Autodesk Fusion 360 part; units mm, degrees
(part 4 of 25)
  arc A1244 (33.5788, 10.6144) -> (33.6296, 10.6144) centre (33.6042, 10.6144) ccw
  arc A1245 (33.2147, 10.8994) -> (33.2147, 10.8486) centre (33.2147, 10.874) ccw
  arc A1246 (32.4278, 11.3271) -> (32.4438, 11.2789) centre (32.4358, 11.303) ccw
  line L381 (32.4358, 10.2249) -> (32.4358, 10.874)
  line L382 (35.6898, 8.9408) -> (35.6898, 9.7197)
  line L383 (32.4358, 11.303) -> (33.6042, 11.6925)
  line L384 (32.9551, 10.2249) -> (32.4358, 10.2249)
  arc A1247 (35.7547, 10.8994) -> (35.7547, 10.8486) centre (35.7547, 10.874) ccw
  arc A1248 (36.0793, 9.3049) -> (36.0793, 9.3557) centre (36.0793, 9.3303) ccw
  arc A1249 (35.8846, 10.8486) -> (35.8846, 10.8994) centre (35.8846, 10.874) ccw
  line L385 (33.3446, 10.874) -> (33.2147, 10.874)
  arc A1250 (32.9805, 10.6144) -> (32.9297, 10.6144) centre (32.9551, 10.6144) ccw
  arc A1251 (32.4358, 10.2503) -> (32.4358, 10.1995) centre (32.4358, 10.2249) ccw
  line L386 (55.2958, 13.5292) -> (55.2958, 13.7889)
  arc A1252 (33.5393, 9.3049) -> (33.5393, 9.3557) centre (33.5393, 9.3303) ccw
  arc A1253 (55.5554, 13.295) -> (55.5554, 13.2442) centre (55.5554, 13.2696) ccw
  arc A1254 (33.2147, 10.8486) -> (33.2147, 10.8994) centre (33.2147, 10.874) ccw
  arc A1255 (33.2147, 10.874) -> (32.9551, 10.6144) centre (33.2147, 10.6144) ccw
  arc A1256 (33.3446, 10.8994) -> (33.3446, 10.8486) centre (33.3446, 10.874) ccw
  arc A1257 (35.7152, 9.7197) -> (35.6644, 9.7197) centre (35.6898, 9.7197) ccw
  line L387 (55.2958, 14.2658) -> (56.4642, 14.2658)
  arc A1258 (32.4612, 10.874) -> (32.4104, 10.874) centre (32.4358, 10.874) ccw
  arc A1259 (55.2958, 14.2912) -> (55.2958, 14.2404) centre (55.2958, 14.2658) ccw
  arc A1260 (33.6122, 11.6684) -> (33.5962, 11.7166) centre (33.6042, 11.6925) ccw
  arc A1261 (32.4104, 10.2249) -> (32.4612, 10.2249) centre (32.4358, 10.2249) ccw
  arc A1262 (33.5962, 11.6684) -> (33.6122, 11.7166) centre (33.6042, 11.6925) ccw
  arc A1263 (55.3212, 13.7889) -> (55.2704, 13.7889) centre (55.2958, 13.7889) ccw
  arc A1264 (36.1188, 10.6144) -> (36.1696, 10.6144) centre (36.1442, 10.6144) ccw
  arc A1265 (55.2958, 13.5292) -> (55.5554, 13.2696) centre (55.5554, 13.5292) ccw
  arc A1266 (33.6296, 10.6144) -> (33.5788, 10.6144) centre (33.6042, 10.6144) ccw
  arc A1267 (33.3446, 10.8486) -> (33.3446, 10.8994) centre (33.3446, 10.874) ccw
  arc A1268 (32.9297, 10.6144) -> (32.9805, 10.6144) centre (32.9551, 10.6144) ccw
  arc A1269 (36.1442, 10.6144) -> (35.8846, 10.874) centre (35.8846, 10.6144) ccw
  arc A1270 (36.1188, 10.2249) -> (36.1696, 10.2249) centre (36.1442, 10.2249) ccw
  arc A1271 (55.5554, 13.2442) -> (55.5554, 13.295) centre (55.5554, 13.2696) ccw
  arc A1272 (33.6042, 10.6144) -> (33.3446, 10.874) centre (33.3446, 10.6144) ccw
  arc A1273 (32.7604, 9.3557) -> (32.7604, 9.3049) centre (32.7604, 9.3303) ccw
  arc A1274 (35.8846, 10.8994) -> (35.8846, 10.8486) centre (35.8846, 10.874) ccw
  line L388 (35.4951, 10.6144) -> (35.4951, 10.2249)
  line L389 (34.9758, 10.2249) -> (34.9758, 10.874)
  arc A1275 (37.5412, 9.2004) -> (37.4904, 9.2004) centre (37.5158, 9.2004) ccw
  arc A1276 (37.5412, 9.5899) -> (37.4904, 9.5899) centre (37.5158, 9.5899) ccw
  arc A1277 (37.8404, 12.0283) -> (37.5158, 11.7037) centre (37.8404, 11.7037) ccw
  arc A1278 (35.4697, 10.2249) -> (35.5205, 10.2249) centre (35.4951, 10.2249) ccw
  arc A1279 (35.5205, 10.6144) -> (35.4697, 10.6144) centre (35.4951, 10.6144) ccw
  line L390 (38.0351, 9.5899) -> (38.6842, 9.5899)
  arc A1280 (38.0351, 9.6153) -> (38.0351, 9.5645) centre (38.0351, 9.5899) ccw
  arc A1281 (38.6842, 10.1346) -> (38.6842, 10.1854) centre (38.6842, 10.16) ccw
  line L391 (38.6842, 9.5899) -> (38.6842, 9.2004)
  arc A1282 (37.5158, 11.4046) -> (37.5158, 11.3538) centre (37.5158, 11.3792) ccw
  arc A1283 (38.6842, 11.7037) -> (38.3596, 12.0283) centre (38.3596, 11.7037) ccw
  arc A1284 (38.3596, 12.0029) -> (38.3596, 12.0537) centre (38.3596, 12.0283) ccw
  line L392 (37.5158, 9.2004) -> (37.5158, 9.5899)
  line L393 (37.5158, 10.16) -> (38.6842, 10.8091)
  arc A1285 (38.0097, 9.3952) -> (38.0605, 9.3952) centre (38.0351, 9.3952) ccw
  arc A1286 (34.9504, 10.2249) -> (35.0012, 10.2249) centre (34.9758, 10.2249) ccw
  arc A1287 (38.0605, 9.5899) -> (38.0097, 9.5899) centre (38.0351, 9.5899) ccw
  arc A1288 (37.5035, 10.1822) -> (37.5281, 10.1378) centre (37.5158, 10.16) ccw
  arc A1289 (35.7547, 10.874) -> (35.4951, 10.6144) centre (35.7547, 10.6144) ccw
  arc A1290 (36.1522, 11.6684) -> (36.1362, 11.7166) centre (36.1442, 11.6925) ccw
  arc A1291 (34.9838, 12.106) -> (34.9678, 12.0578) centre (34.9758, 12.0819) ccw
  arc A1292 (37.5158, 10.8345) -> (37.5158, 10.7837) centre (37.5158, 10.8091) ccw
  arc A1293 (38.4246, 8.9408) -> (38.6842, 9.2004) centre (38.4246, 9.2004) ccw
  arc A1294 (37.4904, 9.2004) -> (37.5412, 9.2004) centre (37.5158, 9.2004) ccw
  arc A1295 (38.6842, 10.7837) -> (38.6842, 10.8345) centre (38.6842, 10.8091) ccw
  arc A1296 (38.6842, 9.5645) -> (38.6842, 9.6153) centre (38.6842, 9.5899) ccw
  arc A1297 (37.5158, 10.1854) -> (37.5158, 10.1346) centre (37.5158, 10.16) ccw
  arc A1298 (38.6965, 10.7869) -> (38.6719, 10.8313) centre (38.6842, 10.8091) ccw
  line L394 (34.9758, 11.303) -> (36.1442, 11.6925)
  arc A1299 (34.9678, 11.3271) -> (34.9838, 11.2789) centre (34.9758, 11.303) ccw
  arc A1300 (37.7754, 8.9154) -> (37.7754, 8.9662) centre (37.7754, 8.9408) ccw
  arc A1301 (35.4697, 10.6144) -> (35.5205, 10.6144) centre (35.4951, 10.6144) ccw
  arc A1302 (38.7096, 9.5899) -> (38.6588, 9.5899) centre (38.6842, 9.5899) ccw
  arc A1303 (38.4246, 8.9154) -> (38.4246, 8.9662) centre (38.4246, 8.9408) ccw
  arc A1304 (37.7754, 8.9662) -> (37.7754, 8.9154) centre (37.7754, 8.9408) ccw
  line L395 (37.5158, 11.3792) -> (37.5158, 11.7037)
  line L396 (38.6842, 10.8091) -> (37.5158, 10.8091)
  arc A1305 (35.4951, 10.1995) -> (35.4951, 10.2503) centre (35.4951, 10.2249) ccw
  line L397 (38.6842, 10.16) -> (37.5158, 10.16)
  line L398 (38.0351, 9.3952) -> (38.0351, 9.5899)
  arc A1306 (35.0012, 10.874) -> (34.9504, 10.874) centre (34.9758, 10.874) ccw
  arc A1307 (37.4904, 11.3792) -> (37.5412, 11.3792) centre (37.5158, 11.3792) ccw
  arc A1308 (37.5158, 9.2004) -> (37.7754, 8.9408) centre (37.7754, 9.2004) ccw
  arc A1309 (37.8404, 12.0029) -> (37.8404, 12.0537) centre (37.8404, 12.0283) ccw
  arc A1310 (37.5412, 11.7037) -> (37.4904, 11.7037) centre (37.5158, 11.7037) ccw
  arc A1311 (34.9758, 10.2503) -> (34.9758, 10.1995) centre (34.9758, 10.2249) ccw
  arc A1312 (38.7096, 9.2004) -> (38.6588, 9.2004) centre (38.6842, 9.2004) ccw
  arc A1313 (38.6842, 11.3538) -> (38.6842, 11.4046) centre (38.6842, 11.3792) ccw
  arc A1314 (37.4904, 11.7037) -> (37.5412, 11.7037) centre (37.5158, 11.7037) ccw
  line L399 (37.8404, 12.0283) -> (38.3596, 12.0283)
  arc A1315 (38.6588, 11.7037) -> (38.7096, 11.7037) centre (38.6842, 11.7037) ccw
  arc A1316 (38.6588, 11.3792) -> (38.7096, 11.3792) centre (38.6842, 11.3792) ccw
  line L400 (29.1451, 28.6399) -> (29.7942, 28.6399)
  line L401 (36.1442, 11.6925) -> (34.9758, 12.0819)
  arc A1317 (38.3596, 12.0537) -> (38.3596, 12.0029) centre (38.3596, 12.0283) ccw
  line L402 (38.6842, 11.3792) -> (37.5158, 11.3792)
  arc A1318 (37.8404, 12.0537) -> (37.8404, 12.0029) centre (37.8404, 12.0283) ccw
  arc A1319 (36.1362, 11.6684) -> (36.1522, 11.7166) centre (36.1442, 11.6925) ccw
  arc A1320 (38.6588, 9.2004) -> (38.7096, 9.2004) centre (38.6842, 9.2004) ccw
  line L403 (35.4951, 10.2249) -> (34.9758, 10.2249)
  arc A1321 (38.4246, 8.9662) -> (38.4246, 8.9154) centre (38.4246, 8.9408) ccw
  line L404 (38.4246, 8.9408) -> (37.7754, 8.9408)
  arc A1322 (51.1175, 9.6224) -> (51.0667, 9.6224) centre (51.0921, 9.6224) ccw
  arc A1323 (48.2115, 10.7198) -> (48.1786, 10.6811) centre (48.1951, 10.7005) ccw
  arc A1324 (50.1904, 10.5382) -> (50.2412, 10.5382) centre (50.2158, 10.5382) ccw
  arc A1325 (48.1951, 10.7005) -> (47.9679, 10.7978) centre (47.968, 10.4841) ccw
  arc A1326 (50.7605, 10.5382) -> (50.7097, 10.5382) centre (50.7351, 10.5382) ccw
  arc A1327 (50.7097, 10.2785) -> (50.7605, 10.2785) centre (50.7351, 10.2785) ccw
  line L405 (53.9242, 8.9408) -> (52.7558, 9.3303)
  arc A1328 (47.9679, 10.8232) -> (47.9679, 10.7724) centre (47.9679, 10.7978) ccw
  arc A1329 (48.1767, 10.6829) -> (48.2135, 10.718) centre (48.1951, 10.7005) ccw
  arc A1330 (48.8277, 10.1294) -> (48.8607, 10.1681) centre (48.8442, 10.1488) ccw
  line L406 (51.3842, 8.9408) -> (50.2158, 9.3303)
  line L407 (48.8442, 10.1487) -> (48.8442, 10.7978)
  arc A1331 (51.4096, 10.4733) -> (51.3588, 10.4733) centre (51.3842, 10.4733) ccw
  arc A1332 (53.9322, 9.6956) -> (53.9162, 9.7438) centre (53.9242, 9.7197) ccw
  arc A1333 (53.6575, 9.6224) -> (53.6067, 9.6224) centre (53.6321, 9.6224) ccw
  line L408 (53.6646, 10.1487) -> (53.6646, 10.7978)
  line L409 (52.7558, 10.4084) -> (53.6646, 10.1487)
  arc A1334 (51.3588, 10.1487) -> (51.4096, 10.1487) centre (51.3842, 10.1487) ccw
  line L410 (50.2158, 10.1487) -> (50.2158, 10.5382)
  arc A1335 (53.6576, 10.1243) -> (53.6715, 10.1731) centre (53.6646, 10.1487) ccw
  arc A1336 (48.8188, 10.1487) -> (48.8696, 10.1487) centre (48.8442, 10.1487) ccw
  line L411 (50.7351, 10.5382) -> (50.7351, 10.2785)
  arc A1337 (53.9162, 8.9167) -> (53.9322, 8.9649) centre (53.9242, 8.9408) ccw
  arc A1338 (50.7097, 10.5382) -> (50.7605, 10.5382) centre (50.7351, 10.5382) ccw
  line L412 (52.7558, 9.3303) -> (53.9242, 9.7197)
  arc A1339 (51.3842, 10.4733) -> (50.7351, 10.4733) centre (51.0597, 10.4733) ccw
  line L413 (48.1951, 10.7005) -> (48.8442, 10.1487)
  arc A1340 (48.8696, 10.7978) -> (48.8188, 10.7978) centre (48.8442, 10.7978) ccw
  arc A1341 (50.2078, 9.3544) -> (50.2238, 9.3062) centre (50.2158, 9.3303) ccw
  arc A1342 (50.7351, 10.5382) -> (50.2158, 10.5382) centre (50.4755, 10.5382) ccw
  line L414 (38.6842, 11.7037) -> (38.6842, 11.3792)
  arc A1343 (51.3762, 8.9167) -> (51.3922, 8.9649) centre (51.3842, 8.9408) ccw
  arc A1344 (51.3588, 10.4733) -> (51.4096, 10.4733) centre (51.3842, 10.4733) ccw
  arc A1345 (52.7638, 9.3544) -> (52.7478, 9.3062) centre (52.7558, 9.3303) ccw
  arc A1346 (50.1904, 10.1487) -> (50.2412, 10.1487) centre (50.2158, 10.1487) ccw
  arc A1347 (52.7478, 9.3544) -> (52.7638, 9.3062) centre (52.7558, 9.3303) ccw
  arc A1348 (51.3922, 9.6956) -> (51.3762, 9.7438) centre (51.3842, 9.7197) ccw
  line L415 (53.6321, 9.6224) -> (53.6321, 9.0382)
  arc A1349 (53.6067, 9.0382) -> (53.6575, 9.0382) centre (53.6321, 9.0382) ccw
  arc A1350 (50.7097, 10.4733) -> (50.7605, 10.4733) centre (50.7351, 10.4733) ccw
  arc A1351 (29.1451, 28.6653) -> (29.1451, 28.6145) centre (29.1451, 28.6399) ccw
  arc A1352 (47.7012, 10.5057) -> (47.6504, 10.5057) centre (47.6758, 10.5057) ccw
  arc A1353 (47.9276, 10.1245) -> (47.9433, 10.1729) centre (47.9355, 10.1487) ccw
  line L416 (51.0921, 9.6224) -> (51.0921, 9.0382)
  arc A1354 (51.0667, 9.0382) -> (51.1175, 9.0382) centre (51.0921, 9.0382) ccw
  arc A1355 (50.2238, 9.3544) -> (50.2078, 9.3062) centre (50.2158, 9.3303) ccw
  arc A1356 (47.6758, 10.5057) -> (47.9354, 10.1487) centre (48.051, 10.5057) ccw
  arc A1357 (29.5346, 27.9908) -> (29.7942, 28.2504) centre (29.5346, 28.2504) ccw
  line L417 (50.2158, 9.3303) -> (51.3842, 9.7197)
  arc A1358 (47.6504, 10.5057) -> (47.7012, 10.5057) centre (47.6758, 10.5057) ccw
  line L418 (51.3842, 10.1487) -> (51.3842, 10.4733)
  arc A1359 (50.2412, 10.5382) -> (50.1904, 10.5382) centre (50.2158, 10.5382) ccw
  arc A1360 (27.3304, 20.6657) -> (27.3812, 20.6657) centre (27.3558, 20.6657) ccw
  arc A1361 (41.2242, 20.2946) -> (41.2242, 20.3454) centre (41.2242, 20.32) ccw
  line L419 (40.5751, 19.7499) -> (41.2242, 19.7499)
  line L420 (25.9842, 19.1008) -> (24.8158, 19.4903)
  arc A1362 (23.0547, 21.034) -> (22.7951, 20.7744) centre (23.0547, 20.7744) ccw
  arc A1363 (27.6479, 20.9324) -> (27.6479, 20.9832) centre (27.6479, 20.9578) ccw
  arc A1364 (27.8915, 20.8798) -> (27.8586, 20.8411) centre (27.8751, 20.8605) ccw
  arc A1365 (40.3804, 22.2137) -> (40.3804, 22.1629) centre (40.3804, 22.1883) ccw
  line L421 (25.0754, 20.3087) -> (24.8158, 20.6333)
  arc A1366 (41.1988, 21.5392) -> (41.2496, 21.5392) centre (41.2242, 21.5392) ccw
  arc A1367 (41.2242, 21.5138) -> (41.2242, 21.5646) centre (41.2242, 21.5392) ccw
  line L422 (31.0642, 19.1008) -> (29.8958, 19.4903)
  arc A1368 (41.2242, 21.8637) -> (40.8996, 22.1883) centre (40.8996, 21.8637) ccw
  arc A1369 (25.9588, 20.3087) -> (26.0096, 20.3087) centre (25.9842, 20.3087) ccw
  arc A1370 (40.0558, 21.5646) -> (40.0558, 21.5138) centre (40.0558, 21.5392) ccw
  arc A1371 (40.0304, 21.8637) -> (40.0812, 21.8637) centre (40.0558, 21.8637) ccw
  line L423 (28.5242, 20.3087) -> (28.5242, 20.9578)
  arc A1372 (24.8078, 19.5144) -> (24.8238, 19.4662) centre (24.8158, 19.4903) ccw
  line L424 (22.7951, 20.7744) -> (22.7951, 20.3849)
  arc A1373 (25.9842, 20.6079) -> (25.9842, 20.6587) centre (25.9842, 20.6333) ccw
  arc A1374 (27.3812, 20.6657) -> (27.3304, 20.6657) centre (27.3558, 20.6657) ccw
  arc A1375 (29.9038, 19.5144) -> (29.8878, 19.4662) centre (29.8958, 19.4903) ccw
  arc A1376 (25.9922, 19.8556) -> (25.9762, 19.9038) centre (25.9842, 19.8797) ccw
  arc A1377 (28.4988, 20.3087) -> (28.5496, 20.3087) centre (28.5242, 20.3087) ccw
  arc A1378 (28.5162, 19.0767) -> (28.5322, 19.1249) centre (28.5242, 19.1008) ccw
  arc A1379 (40.0558, 20.3454) -> (40.0558, 20.2946) centre (40.0558, 20.32) ccw
  arc A1380 (28.5322, 19.8556) -> (28.5162, 19.9038) centre (28.5242, 19.8797) ccw
  arc A1381 (27.8567, 20.8429) -> (27.8935, 20.878) centre (27.8751, 20.8605) ccw
  arc A1382 (41.1988, 21.8637) -> (41.2496, 21.8637) centre (41.2242, 21.8637) ccw
  line L425 (25.6921, 19.7824) -> (25.6921, 19.1982)
  arc A1383 (41.2242, 20.9437) -> (41.2242, 20.9945) centre (41.2242, 20.9691) ccw
  arc A1384 (25.9762, 19.0767) -> (25.9922, 19.1249) centre (25.9842, 19.1008) ccw
  arc A1385 (24.8238, 19.5144) -> (24.8078, 19.4662) centre (24.8158, 19.4903) ccw
  arc A1386 (40.8996, 22.2137) -> (40.8996, 22.1629) centre (40.8996, 22.1883) ccw
  arc A1387 (23.0547, 21.0086) -> (23.0547, 21.0594) centre (23.0547, 21.034) ccw
  arc A1388 (27.6479, 20.9832) -> (27.6479, 20.9324) centre (27.6479, 20.9578) ccw
  arc A1389 (28.2067, 19.1982) -> (28.2575, 19.1982) centre (28.2321, 19.1982) ccw
  arc A1390 (41.2496, 21.8637) -> (41.1988, 21.8637) centre (41.2242, 21.8637) ccw
  arc A1391 (25.7175, 19.7824) -> (25.6667, 19.7824) centre (25.6921, 19.7824) ccw
  line L426 (27.8751, 20.8605) -> (28.5242, 20.3087)
  arc A1392 (28.5077, 20.2894) -> (28.5407, 20.3281) centre (28.5242, 20.3087) ccw
  arc A1393 (28.2575, 19.7824) -> (28.2067, 19.7824) centre (28.2321, 19.7824) ccw
  arc A1394 (31.0562, 19.0767) -> (31.0722, 19.1249) centre (31.0642, 19.1008) ccw
  arc A1395 (25.0556, 20.2928) -> (25.0953, 20.3246) centre (25.0755, 20.3087) ccw
  arc A1396 (23.3793, 19.4649) -> (23.3793, 19.5157) centre (23.3793, 19.4903) ccw
  line L427 (24.8158, 20.6333) -> (25.9842, 20.6333)
  line L428 (25.9842, 20.3087) -> (25.9842, 20.9578)
  arc A1397 (40.3804, 22.1629) -> (40.3804, 22.2137) centre (40.3804, 22.1883) ccw
  arc A1398 (24.8158, 20.6587) -> (24.8158, 20.6079) centre (24.8158, 20.6333) ccw
  line L429 (28.5242, 19.1008) -> (27.3558, 19.4903)
  arc A1399 (23.0152, 19.8797) -> (22.9644, 19.8797) centre (22.9898, 19.8797) ccw
  line L430 (41.2242, 21.5392) -> (40.0558, 21.5392)
  arc A1400 (27.3638, 19.5144) -> (27.3478, 19.4662) centre (27.3558, 19.4903) ccw
  arc A1401 (40.0812, 21.8637) -> (40.0304, 21.8637) centre (40.0558, 21.8637) ccw
  line L431 (40.3804, 22.1883) -> (40.8996, 22.1883)
  arc A1402 (25.6667, 19.1982) -> (25.7175, 19.1982) centre (25.6921, 19.1982) ccw
  arc A1403 (24.8356, 20.6491) -> (24.796, 20.6174) centre (24.8158, 20.6333) ccw
  line L432 (27.3558, 19.4903) -> (28.5242, 19.8797)
  arc A1404 (41.2365, 20.9469) -> (41.2119, 20.9913) centre (41.2242, 20.9691) ccw
  arc A1405 (26.0096, 20.9578) -> (25.9588, 20.9578) centre (25.9842, 20.9578) ccw
  line L433 (28.2321, 19.7824) -> (28.2321, 19.1982)
  arc A1406 (27.8751, 20.8605) -> (27.6479, 20.9578) centre (27.648, 20.6441) ccw
  line L434 (24.8158, 19.4903) -> (25.9842, 19.8797)
  arc A1407 (27.6479, 20.9578) -> (27.3558, 20.6657) centre (27.6479, 20.6657) ccw
  line L435 (32.7604, 20.931) -> (33.0849, 20.931)
  arc A1408 (32.7604, 20.9564) -> (32.7604, 20.9056) centre (32.7604, 20.931) ccw
  arc A1409 (31.0896, 20.6333) -> (31.0388, 20.6333) centre (31.0642, 20.6333) ccw
  arc A1410 (32.7604, 20.2565) -> (32.7604, 20.3073) centre (32.7604, 20.2819) ccw
  arc A1411 (33.6042, 20.4117) -> (33.0849, 20.931) centre (33.0849, 20.4117) ccw
  arc A1412 (30.3897, 20.4385) -> (30.4405, 20.4385) centre (30.4151, 20.4385) ccw
  arc A1413 (32.4612, 19.4254) -> (32.4104, 19.4254) centre (32.4358, 19.4254) ccw
  arc A1414 (40.3804, 22.1883) -> (40.0558, 21.8637) centre (40.3804, 21.8637) ccw
  arc A1415 (27.6076, 20.2845) -> (27.6233, 20.3329) centre (27.6155, 20.3087) ccw
  arc A1416 (35.3004, 19.7499) -> (34.9758, 19.4254) centre (35.3004, 19.4253) ccw
  arc A1417 (34.9504, 19.1008) -> (35.0012, 19.1008) centre (34.9758, 19.1008) ccw
  arc A1418 (30.7467, 19.1982) -> (30.7975, 19.1982) centre (30.7721, 19.1982) ccw
  arc A1419 (40.8996, 22.1629) -> (40.8996, 22.2137) centre (40.8996, 22.1883) ccw
  arc A1420 (27.3478, 19.5144) -> (27.3638, 19.4662) centre (27.3558, 19.4903) ccw
  arc A1421 (32.4358, 19.1262) -> (32.4358, 19.0754) centre (32.4358, 19.1008) ccw
  arc A1422 (32.4104, 19.4254) -> (32.4612, 19.4254) centre (32.4358, 19.4254) ccw
  arc A1423 (32.8253, 20.2819) -> (33.0849, 20.5415) centre (32.8253, 20.5415) ccw
  line L436 (33.6042, 19.1008) -> (32.4358, 19.1008)
  arc A1424 (29.8878, 19.5144) -> (29.9038, 19.4662) centre (29.8958, 19.4903) ccw
  arc A1425 (32.8253, 20.3073) -> (32.8253, 20.2565) centre (32.8253, 20.2819) ccw
  arc A1426 (33.1103, 20.5415) -> (33.0595, 20.5415) centre (33.0849, 20.5415) ccw
  arc A1427 (32.8253, 20.2565) -> (32.8253, 20.3073) centre (32.8253, 20.2819) ccw
  line L437 (40.0558, 21.5392) -> (40.0558, 21.8637)
  arc A1428 (31.0642, 20.6333) -> (30.4151, 20.6333) centre (30.7396, 20.6333) ccw
  line L438 (31.0642, 20.3087) -> (31.0642, 20.6333)
  line L439 (33.6042, 19.4254) -> (33.6042, 19.1008)
  arc A1429 (27.3558, 20.6657) -> (27.6154, 20.3087) centre (27.731, 20.6657) ccw
  line L440 (41.2242, 21.8637) -> (41.2242, 21.5392)
  line L441 (29.8958, 19.4903) -> (31.0642, 19.8797)
  line L442 (30.4151, 20.6982) -> (30.4151, 20.4385)
  arc A1430 (31.0388, 20.6333) -> (31.0896, 20.6333) centre (31.0642, 20.6333) ccw
  arc A1431 (30.4405, 20.6982) -> (30.3897, 20.6982) centre (30.4151, 20.6982) ccw
  arc A1432 (33.6042, 19.4254) -> (33.2796, 19.7499) centre (33.2796, 19.4253) ccw
  arc A1433 (33.0595, 20.5415) -> (33.1103, 20.5415) centre (33.0849, 20.5415) ccw
  arc A1434 (32.7604, 19.7499) -> (32.4358, 19.4254) centre (32.7604, 19.4253) ccw
  arc A1435 (40.0304, 21.5392) -> (40.0812, 21.5392) centre (40.0558, 21.5392) ccw
  arc A1436 (30.4151, 20.6982) -> (29.8958, 20.6982) centre (30.1554, 20.6982) ccw
  arc A1437 (32.7604, 20.3073) -> (32.7604, 20.2565) centre (32.7604, 20.2819) ccw
  line L443 (32.7604, 19.7499) -> (33.2796, 19.7499)
  arc A1438 (33.5788, 19.1008) -> (33.6296, 19.1008) centre (33.6042, 19.1008) ccw
  line L444 (34.9758, 19.1008) -> (34.9758, 19.4254)
  arc A1439 (31.0722, 19.8556) -> (31.0562, 19.9038) centre (31.0642, 19.8797) ccw
  arc A1440 (30.3897, 20.6982) -> (30.4405, 20.6982) centre (30.4151, 20.6982) ccw
  arc A1441 (28.5496, 20.9578) -> (28.4988, 20.9578) centre (28.5242, 20.9578) ccw
  arc A1442 (33.2796, 19.7753) -> (33.2796, 19.7245) centre (33.2796, 19.7499) ccw
  arc A1443 (29.8704, 20.6982) -> (29.9212, 20.6982) centre (29.8958, 20.6982) ccw
  arc A1444 (32.4104, 19.1008) -> (32.4612, 19.1008) centre (32.4358, 19.1008) ccw
  arc A1445 (32.7604, 19.7245) -> (32.7604, 19.7753) centre (32.7604, 19.7499) ccw
  arc A1446 (33.0849, 20.9056) -> (33.0849, 20.9564) centre (33.0849, 20.931) ccw
  arc A1447 (29.8704, 20.3087) -> (29.9212, 20.3087) centre (29.8958, 20.3087) ccw
  arc A1448 (32.7604, 19.7753) -> (32.7604, 19.7245) centre (32.7604, 19.7499) ccw
  arc A1449 (30.7975, 19.7824) -> (30.7467, 19.7824) centre (30.7721, 19.7824) ccw
  line L445 (29.8958, 20.3087) -> (29.8958, 20.6982)
  line L446 (30.7721, 19.7824) -> (30.7721, 19.1982)
  arc A1450 (33.2796, 19.7245) -> (33.2796, 19.7753) centre (33.2796, 19.7499) ccw
  arc A1451 (31.0388, 20.3087) -> (31.0896, 20.3087) centre (31.0642, 20.3087) ccw
  arc A1452 (30.3897, 20.6333) -> (30.4405, 20.6333) centre (30.4151, 20.6333) ccw
  arc A1453 (32.7604, 20.931) -> (32.7604, 20.2819) centre (32.7604, 20.6065) ccw
  arc A1454 (35.0012, 19.4254) -> (34.9504, 19.4254) centre (34.9758, 19.4254) ccw
  line L447 (33.0849, 20.931) -> (33.0849, 20.5415)
  arc A1455 (29.9212, 20.6982) -> (29.8704, 20.6982) centre (29.8958, 20.6982) ccw
  line L448 (32.4358, 19.1008) -> (32.4358, 19.4254)
  arc A1456 (32.7604, 20.9056) -> (32.7604, 20.9564) centre (32.7604, 20.931) ccw
  arc A1457 (33.6296, 19.4254) -> (33.5788, 19.4254) centre (33.6042, 19.4254) ccw
  line L449 (36.1442, 20.2819) -> (36.1442, 20.931)
  arc A1458 (35.1269, 21.9995) -> (35.1492, 21.9538) centre (35.138, 21.9767) ccw
  arc A1459 (34.9956, 20.6223) -> (34.956, 20.5906) centre (34.9758, 20.6065) ccw
  arc A1460 (35.2513, 22.0289) -> (35.2196, 21.9893) centre (35.2355, 22.0091) ccw
  arc A1461 (35.1492, 21.5451) -> (35.1269, 21.4994) centre (35.138, 21.5223) ccw
  arc A1462 (35.9737, 21.5463) -> (35.9902, 21.4982) centre (35.9819, 21.5222) ccw
  arc A1463 (35.9902, 22.0007) -> (35.9737, 21.9526) centre (35.9819, 21.9767) ccw
  arc A1464 (38.2552, 25.0613) -> (38.2044, 25.0613) centre (38.2298, 25.0613) ccw
  line L450 (36.1442, 19.4254) -> (36.1442, 19.1008)
  arc A1465 (33.1103, 20.931) -> (33.0595, 20.931) centre (33.0849, 20.931) ccw
  arc A1466 (36.1188, 19.1008) -> (36.1696, 19.1008) centre (36.1442, 19.1008) ccw
  arc A1467 (35.8196, 19.7753) -> (35.8196, 19.7245) centre (35.8196, 19.7499) ccw
  arc A1468 (38.2552, 23.7659) -> (38.2044, 23.7659) centre (38.2298, 23.7659) ccw
  line L451 (38.2298, 24.2824) -> (38.2298, 25.0613)
  arc A1469 (33.5788, 19.4254) -> (33.6296, 19.4254) centre (33.6042, 19.4254) ccw
  arc A1470 (34.9758, 19.1262) -> (34.9758, 19.0754) centre (34.9758, 19.1008) ccw
  arc A1471 (36.1442, 19.0754) -> (36.1442, 19.1262) centre (36.1442, 19.1008) ccw
  line L452 (38.2298, 20.3962) -> (38.2298, 21.1751)
  line L453 (35.3004, 19.7499) -> (35.8196, 19.7499)
  arc A1472 (35.56, 21.4503) -> (35.56, 21.3995) centre (35.56, 21.4249) ccw
  arc A1473 (36.1188, 20.2819) -> (36.1696, 20.2819) centre (36.1442, 20.2819) ccw
  arc A1474 (35.8687, 21.47) -> (35.9004, 21.5096) centre (35.8845, 21.4898) ccw
  arc A1475 (38.2552, 19.8797) -> (38.2044, 19.8797) centre (38.2298, 19.8797) ccw
  arc A1476 (38.2044, 24.2824) -> (38.2552, 24.2824) centre (38.2298, 24.2824) ccw
  line L454 (38.2298, 22.987) -> (38.2298, 23.7659)
  arc A1477 (33.0849, 20.9564) -> (33.0849, 20.9056) centre (33.0849, 20.931) ccw
  arc A1478 (35.56, 22.074) -> (35.1381, 21.9766) centre (35.5601, 21.1113) ccw
  arc A1479 (35.0012, 21.7494) -> (34.9504, 21.7494) centre (34.9758, 21.7494) ccw
  arc A1480 (33.6042, 19.0754) -> (33.6042, 19.1262) centre (33.6042, 19.1008) ccw
  arc A1481 (34.9758, 20.6319) -> (34.9758, 20.5811) centre (34.9758, 20.6065) ccw
  arc A1482 (33.5788, 20.4117) -> (33.6296, 20.4117) centre (33.6042, 20.4117) ccw
  line L455 (34.9758, 20.6065) -> (36.1442, 20.6065)
  arc A1483 (34.9504, 21.7494) -> (35.0012, 21.7494) centre (34.9758, 21.7494) ccw
  arc A1484 (38.2044, 20.3962) -> (38.2552, 20.3962) centre (38.2298, 20.3962) ccw
  arc A1485 (36.1442, 21.7494) -> (35.9819, 21.9766) centre (35.904, 21.7494) ccw
  arc A1486 (35.1381, 21.9766) -> (34.9758, 21.7494) centre (35.216, 21.7494) ccw
  arc A1487 (36.1696, 21.7494) -> (36.1188, 21.7494) centre (36.1442, 21.7494) ccw
  arc A1488 (36.1442, 20.5811) -> (36.1442, 20.6319) centre (36.1442, 20.6065) ccw
  arc A1489 (35.1463, 21.9526) -> (35.1298, 22.0007) centre (35.138, 21.9766) ccw
  arc A1490 (35.9931, 21.4994) -> (35.9708, 21.5451) centre (35.982, 21.5223) ccw
  line L456 (32.8253, 20.2819) -> (32.7604, 20.2819)
  arc A1491 (35.56, 21.4249) -> (35.9819, 21.5223) centre (35.5599, 22.3876) ccw
  arc A1492 (36.1442, 19.4254) -> (35.8196, 19.7499) centre (35.8196, 19.4253) ccw
  arc A1493 (35.3004, 19.7753) -> (35.3004, 19.7245) centre (35.3004, 19.7499) ccw
  arc A1494 (35.56, 22.0994) -> (35.56, 22.0486) centre (35.56, 22.074) ccw
  line L457 (38.2298, 19.1008) -> (38.2298, 19.8797)
  arc A1495 (34.9504, 19.4254) -> (35.0012, 19.4254) centre (34.9758, 19.4254) ccw
  arc A1496 (36.1696, 20.931) -> (36.1188, 20.931) centre (36.1442, 20.931) ccw
  line L458 (76.7842, 35.6108) -> (75.6158, 36.0003)
  arc A1497 (35.9819, 21.5223) -> (36.1442, 21.7494) centre (35.9041, 21.7494) ccw
  arc A1498 (35.8196, 19.7245) -> (35.8196, 19.7753) centre (35.8196, 19.7499) ccw
  arc A1499 (36.1188, 21.7494) -> (36.1696, 21.7494) centre (36.1442, 21.7494) ccw
  arc A1500 (35.56, 22.0486) -> (35.56, 22.0994) centre (35.56, 22.074) ccw
  arc A1501 (75.6238, 36.0244) -> (75.6078, 35.9762) centre (75.6158, 36.0003) ccw
  arc A1502 (35.1381, 21.5223) -> (35.56, 21.4249) centre (35.5601, 22.3876) ccw
  arc A1503 (34.9758, 21.7494) -> (35.1381, 21.5223) centre (35.2159, 21.7494) ccw
  arc A1504 (35.1298, 21.4982) -> (35.1463, 21.5463) centre (35.1381, 21.5222) ccw
  line L459 (38.2298, 21.6916) -> (38.2298, 22.4705)
  arc A1505 (35.9819, 21.9766) -> (35.56, 22.074) centre (35.5599, 21.1113) ccw
  arc A1506 (36.1696, 19.4254) -> (36.1188, 19.4254) centre (36.1442, 19.4254) ccw
  arc A1507 (38.2044, 19.1008) -> (38.2552, 19.1008) centre (38.2298, 19.1008) ccw
  arc A1508 (35.9708, 21.9538) -> (35.9931, 21.9995) centre (35.9819, 21.9767) ccw
  arc A1509 (36.1188, 19.4254) -> (36.1696, 19.4254) centre (36.1442, 19.4254) ccw
  line L460 (36.1442, 19.1008) -> (34.9758, 19.1008)
  arc A1510 (75.9404, 40.6301) -> (75.6158, 40.3056) centre (75.9404, 40.3055) ccw
  arc A1511 (75.5904, 40.3056) -> (75.6412, 40.3056) centre (75.6158, 40.3056) ccw
  arc A1512 (75.6228, 37.1028) -> (75.6088, 37.0539) centre (75.6158, 37.0784) ccw
  arc A1513 (75.6412, 40.3056) -> (75.5904, 40.3056) centre (75.6158, 40.3056) ccw
  arc A1514 (75.7335, 39.407) -> (75.6928, 39.4374) centre (75.7132, 39.4222) ccw
  arc A1515 (76.4596, 40.6555) -> (76.4596, 40.6047) centre (76.4596, 40.6301) ccw
  arc A1516 (76.4992, 36.8187) -> (76.55, 36.8187) centre (76.5246, 36.8187) ccw
  arc A1517 (76.2649, 37.2985) -> (76.2649, 37.2477) centre (76.2649, 37.2731) ccw
  line L461 (75.6158, 36.0003) -> (76.7842, 36.3897)
  arc A1518 (75.9404, 40.6047) -> (75.9404, 40.6555) centre (75.9404, 40.6301) ccw
  line L462 (76.914, 37.9123) -> (75.486, 38.4316)
  arc A1519 (76.0803, 39.0124) -> (76.1249, 38.9881) centre (76.1026, 39.0003) ccw
  arc A1520 (38.2552, 21.1751) -> (38.2044, 21.1751) centre (38.2298, 21.1751) ccw
  line L463 (76.2649, 37.2731) -> (76.7842, 37.2731)
  arc A1521 (76.55, 37.4678) -> (76.4992, 37.4678) centre (76.5246, 37.4678) ccw
  arc A1522 (75.6078, 36.0244) -> (75.6238, 35.9762) centre (75.6158, 36.0003) ccw
  arc A1523 (75.8754, 38.8705) -> (76.1026, 39.0003) centre (75.8754, 39.1342) ccw
  arc A1524 (76.7588, 39.2275) -> (76.8096, 39.2275) centre (76.7842, 39.2275) ccw
  arc A1525 (76.8096, 39.2275) -> (76.7588, 39.2275) centre (76.7842, 39.2275) ccw
  arc A1526 (35.3004, 19.7245) -> (35.3004, 19.7753) centre (35.3004, 19.7499) ccw
  line L464 (76.2974, 39.3573) -> (76.1026, 39.0003)
  arc A1527 (38.2044, 21.6916) -> (38.2552, 21.6916) centre (38.2298, 21.6916) ccw
  arc A1528 (76.6219, 38.838) -> (76.7842, 39.2275) centre (76.2357, 39.2275) ccw
  arc A1529 (35.2156, 20.266) -> (35.2553, 20.2978) centre (35.2355, 20.2819) ccw
  arc A1530 (75.8754, 38.8959) -> (75.8754, 38.8451) centre (75.8754, 38.8705) ccw
  line L465 (76.7842, 39.981) -> (75.6158, 39.981)
  line L466 (75.6158, 41.4867) -> (76.7842, 41.8761)
  line L467 (75.6158, 37.0784) -> (76.5246, 36.8187)
  arc A1531 (76.7922, 41.852) -> (76.7762, 41.9002) centre (76.7842, 41.8761) ccw
  arc A1532 (75.4947, 38.4555) -> (75.4773, 38.4077) centre (75.486, 38.4316) ccw
  arc A1533 (75.6158, 39.1301) -> (75.8754, 38.8705) centre (75.8754, 39.1301) ccw
  arc A1534 (76.9053, 37.8884) -> (76.9227, 37.9362) centre (76.914, 37.9123) ccw
  arc A1535 (75.6412, 39.1301) -> (75.5904, 39.1301) centre (75.6158, 39.1301) ccw
  line L468 (35.8846, 21.4898) -> (35.2354, 22.0091)
  arc A1536 (38.2044, 22.987) -> (38.2552, 22.987) centre (38.2298, 22.987) ccw
  arc A1537 (76.4596, 40.6047) -> (76.4596, 40.6555) centre (76.4596, 40.6301) ccw
  arc A1538 (75.6158, 40.0064) -> (75.6158, 39.9556) centre (75.6158, 39.981) ccw
  arc A1539 (35.56, 21.3995) -> (35.56, 21.4503) centre (35.56, 21.4249) ccw
  arc A1540 (76.5246, 39.4871) -> (76.2974, 39.3573) centre (76.5246, 39.2234) ccw
  arc A1541 (76.7842, 39.2275) -> (76.5246, 39.4871) centre (76.5246, 39.2275) ccw
  arc A1542 (76.7922, 36.3656) -> (76.7762, 36.4138) centre (76.7842, 36.3897) ccw
  arc A1543 (75.9404, 40.6555) -> (75.9404, 40.6047) centre (75.9404, 40.6301) ccw
  line L469 (35.2354, 20.2819) -> (34.9758, 20.6065)
  arc A1544 (75.7132, 39.4222) -> (75.6158, 39.1301) centre (76.1026, 39.1301) ccw
  arc A1545 (76.7842, 39.9556) -> (76.7842, 40.0064) centre (76.7842, 39.981) ccw
  arc A1546 (76.7588, 40.3056) -> (76.8096, 40.3056) centre (76.7842, 40.3056) ccw
  arc A1547 (76.2755, 39.3702) -> (76.3193, 39.3444) centre (76.2974, 39.3573) ccw
  line L470 (76.7842, 40.3056) -> (76.7842, 39.981)
  arc A1548 (75.5904, 39.1301) -> (75.6412, 39.1301) centre (75.6158, 39.1301) ccw
  arc A1549 (76.604, 38.856) -> (76.6398, 38.82) centre (76.6219, 38.838) ccw
  line L471 (76.5246, 36.8187) -> (76.5246, 37.4678)
  arc A1550 (76.5246, 39.5125) -> (76.5246, 39.4617) centre (76.5246, 39.4871) ccw
  arc A1551 (76.7842, 37.2477) -> (76.7842, 37.2985) centre (76.7842, 37.2731) ccw
  arc A1552 (75.6078, 41.5108) -> (75.6238, 41.4626) centre (75.6158, 41.4867) ccw
  line L472 (75.6158, 39.981) -> (75.6158, 40.3056)
  line L473 (75.9404, 40.6301) -> (76.4596, 40.6301)
  arc A1553 (38.2552, 22.4705) -> (38.2044, 22.4705) centre (38.2298, 22.4705) ccw
  arc A1554 (75.5904, 39.981) -> (75.6412, 39.981) centre (75.6158, 39.981) ccw
  arc A1555 (76.4667, 35.7082) -> (76.5175, 35.7082) centre (76.4921, 35.7082) ccw
  arc A1556 (76.7762, 35.5867) -> (76.7922, 35.6349) centre (76.7842, 35.6108) ccw
  arc A1557 (76.5176, 36.7943) -> (76.5315, 36.8431) centre (76.5246, 36.8187) ccw
  arc A1558 (76.5175, 36.2924) -> (76.4667, 36.2924) centre (76.4921, 36.2924) ccw
  line L474 (76.4921, 36.2924) -> (76.4921, 35.7082)
  arc A1559 (75.8754, 38.8451) -> (75.8754, 38.8959) centre (75.8754, 38.8705) ccw
  arc A1560 (76.7762, 41.0731) -> (76.7922, 41.1213) centre (76.7842, 41.0972) ccw
  arc A1561 (76.4667, 41.1946) -> (76.5175, 41.1946) centre (76.4921, 41.1946) ccw
  arc A1562 (79.3496, 40.1992) -> (79.2988, 40.1992) centre (79.3242, 40.1992) ccw
  arc A1563 (79.3242, 39.2275) -> (79.0646, 39.4871) centre (79.0646, 39.2275) ccw
  arc A1564 (78.6497, 36.8187) -> (78.7005, 36.8187) centre (78.6751, 36.8187) ccw
  arc A1565 (76.7842, 40.3056) -> (76.4596, 40.6301) centre (76.4596, 40.3055) ccw
  arc A1566 (76.8096, 40.3056) -> (76.7588, 40.3056) centre (76.7842, 40.3056) ccw
  arc A1567 (78.9347, 37.4932) -> (78.9347, 37.4424) centre (78.9347, 37.4678) ccw
  arc A1568 (79.4453, 37.8884) -> (79.4627, 37.9362) centre (79.454, 37.9123) ccw
  arc A1569 (79.0646, 39.965) -> (79.0646, 39.9142) centre (79.0646, 39.9396) ccw
  line L475 (78.1558, 36.8187) -> (78.1558, 37.4678)
  line L476 (79.0321, 36.2924) -> (79.0321, 35.7082)
  arc A1570 (79.3322, 36.3656) -> (79.3162, 36.4138) centre (79.3242, 36.3897) ccw
  arc A1571 (78.9347, 37.4678) -> (78.6751, 37.2082) centre (78.9347, 37.2082) ccw
  arc A1572 (78.6751, 36.7933) -> (78.6751, 36.8441) centre (78.6751, 36.8187) ccw
  arc A1573 (79.0646, 37.4932) -> (79.0646, 37.4424) centre (79.0646, 37.4678) ccw
  arc A1574 (79.2988, 37.2082) -> (79.3496, 37.2082) centre (79.3242, 37.2082) ccw
  line L477 (78.8374, 39.3573) -> (78.6426, 39.0003)
  line L478 (79.3242, 40.4589) -> (79.3242, 40.1992)
  arc A1575 (76.5175, 41.7788) -> (76.4667, 41.7788) centre (76.4921, 41.7788) ccw
  arc A1576 (76.1245, 38.9874) -> (76.0808, 39.0132) centre (76.1026, 39.0003) ccw
  arc A1577 (75.6238, 41.5108) -> (75.6078, 41.4626) centre (75.6158, 41.4867) ccw
  arc A1578 (78.8597, 39.3451) -> (78.8151, 39.3695) centre (78.8374, 39.3573) ccw
  arc A1579 (79.3242, 37.2082) -> (79.0646, 37.4678) centre (79.0646, 37.2082) ccw
  arc A1580 (78.1478, 36.0244) -> (78.1638, 35.9762) centre (78.1558, 36.0003) ccw
  line L479 (78.6751, 36.8187) -> (78.1558, 36.8187)
  line L480 (78.1558, 36.0003) -> (79.3242, 36.3897)
  arc A1581 (78.0347, 38.4555) -> (78.0173, 38.4077) centre (78.026, 38.4316) ccw
  arc A1582 (79.0646, 39.9396) -> (79.3242, 40.1992) centre (79.0646, 40.1992) ccw
  line L481 (79.0646, 37.4678) -> (78.9347, 37.4678)
  arc A1583 (76.5246, 39.4617) -> (76.5246, 39.5125) centre (76.5246, 39.4871) ccw
  arc A1584 (79.1619, 38.838) -> (79.3242, 39.2275) centre (78.7757, 39.2275) ccw
  line L482 (79.0646, 39.9396) -> (78.4154, 39.9396)
  arc A1585 (78.1304, 39.1301) -> (78.1812, 39.1301) centre (78.1558, 39.1301) ccw
  arc A1586 (79.0646, 37.4424) -> (79.0646, 37.4932) centre (79.0646, 37.4678) ccw
  line L483 (76.4921, 41.7788) -> (76.4921, 41.1946)
  arc A1587 (79.144, 38.856) -> (79.1798, 38.82) centre (79.1619, 38.838) ccw
  arc A1588 (79.3162, 35.5867) -> (79.3322, 35.6349) centre (79.3242, 35.6108) ccw
  arc A1589 (78.4154, 38.8451) -> (78.4154, 38.8959) centre (78.4154, 38.8705) ccw
  arc A1590 (76.7588, 39.981) -> (76.8096, 39.981) centre (76.7842, 39.981) ccw
  arc A1591 (79.0575, 36.2924) -> (79.0067, 36.2924) centre (79.0321, 36.2924) ccw
  arc A1592 (78.1304, 36.8187) -> (78.1812, 36.8187) centre (78.1558, 36.8187) ccw
  arc A1593 (78.1812, 39.1301) -> (78.1304, 39.1301) centre (78.1558, 39.1301) ccw
  arc A1594 (79.0646, 39.4617) -> (79.0646, 39.5125) centre (79.0646, 39.4871) ccw
  arc A1595 (79.2988, 40.1992) -> (79.3496, 40.1992) centre (79.3242, 40.1992) ccw
  line L484 (78.6751, 37.2082) -> (78.6751, 36.8187)
  arc A1596 (78.2532, 39.4222) -> (78.1558, 39.1301) centre (78.6426, 39.1301) ccw
  arc A1597 (76.3197, 39.3451) -> (76.2751, 39.3695) centre (76.2974, 39.3573) ccw
  arc A1598 (78.1812, 37.4678) -> (78.1304, 37.4678) centre (78.1558, 37.4678) ccw
  arc A1599 (78.1638, 36.0244) -> (78.1478, 35.9762) centre (78.1558, 36.0003) ccw
  arc A1600 (79.0646, 39.4871) -> (78.8374, 39.3573) centre (79.0646, 39.2234) ccw
  arc A1601 (79.3496, 37.2082) -> (79.2988, 37.2082) centre (79.3242, 37.2082) ccw
  arc A1602 (78.6497, 37.2082) -> (78.7005, 37.2082) centre (78.6751, 37.2082) ccw
  arc A1603 (78.1558, 39.1301) -> (78.4154, 38.8705) centre (78.4154, 39.1301) ccw
  arc A1604 (79.0067, 35.7082) -> (79.0575, 35.7082) centre (79.0321, 35.7082) ccw
  arc A1605 (79.3496, 39.2275) -> (79.2988, 39.2275) centre (79.3242, 39.2275) ccw
  arc A1606 (79.2988, 36.8187) -> (79.3496, 36.8187) centre (79.3242, 36.8187) ccw
  line L485 (79.454, 37.9123) -> (78.026, 38.4316)
  arc A1607 (79.2988, 39.2275) -> (79.3496, 39.2275) centre (79.3242, 39.2275) ccw
  arc A1608 (78.6645, 38.9874) -> (78.6208, 39.0132) centre (78.6427, 39.0003) ccw
  arc A1609 (78.2735, 39.407) -> (78.2328, 39.4374) centre (78.2532, 39.4222) ccw
  line L486 (76.7842, 41.0972) -> (75.6158, 41.4867)
  arc A1610 (78.4154, 38.8705) -> (78.6426, 39.0003) centre (78.4154, 39.1342) ccw
  arc A1611 (78.9347, 37.4424) -> (78.9347, 37.4932) centre (78.9347, 37.4678) ccw
  line L487 (79.3242, 36.8187) -> (79.3242, 37.2082)
  arc A1612 (81.8642, 39.6437) -> (81.5396, 39.9683) centre (81.5396, 39.6437) ccw
  arc A1613 (81.8642, 38.0746) -> (81.8642, 38.1254) centre (81.8642, 38.1) ccw
  arc A1614 (80.6704, 37.1404) -> (80.7212, 37.1404) centre (80.6958, 37.1404) ccw
  arc A1615 (78.7005, 37.2082) -> (78.6497, 37.2082) centre (78.6751, 37.2082) ccw
  arc A1616 (81.8896, 37.1404) -> (81.8388, 37.1404) centre (81.8642, 37.1404) ccw
  line L488 (81.6046, 36.8808) -> (80.9554, 36.8808)
  arc A1617 (81.8896, 37.5299) -> (81.8388, 37.5299) centre (81.8642, 37.5299) ccw
  arc A1618 (81.8642, 39.2938) -> (81.8642, 39.3446) centre (81.8642, 39.3192) ccw
  line L489 (79.3242, 35.6108) -> (78.1558, 36.0003)
  arc A1619 (78.1558, 36.8441) -> (78.1558, 36.7933) centre (78.1558, 36.8187) ccw
  arc A1620 (78.8155, 39.3702) -> (78.8593, 39.3444) centre (78.8374, 39.3573) ccw
  arc A1621 (81.8896, 39.6437) -> (81.8388, 39.6437) centre (81.8642, 39.6437) ccw
  arc A1622 (78.1558, 40.1992) -> (78.4154, 39.9396) centre (78.4154, 40.1992) ccw
  arc A1623 (81.1897, 37.3352) -> (81.2405, 37.3352) centre (81.2151, 37.3352) ccw
  arc A1624 (81.8765, 38.7269) -> (81.8519, 38.7713) centre (81.8642, 38.7491) ccw
  arc A1625 (81.5396, 39.9937) -> (81.5396, 39.9429) centre (81.5396, 39.9683) ccw
  arc A1626 (81.8642, 37.5045) -> (81.8642, 37.5553) centre (81.8642, 37.5299) ccw
  arc A1627 (79.2988, 40.9358) -> (79.3496, 40.9358) centre (79.3242, 40.9358) ccw
  line L490 (78.1558, 40.9358) -> (79.3242, 40.9358)
  arc A1628 (80.6958, 38.7745) -> (80.6958, 38.7237) centre (80.6958, 38.7491) ccw
  arc A1629 (78.1304, 40.1992) -> (78.1812, 40.1992) centre (78.1558, 40.1992) ccw
  arc A1630 (80.7212, 37.1404) -> (80.6704, 37.1404) centre (80.6958, 37.1404) ccw
  line L491 (80.6958, 39.3192) -> (80.6958, 39.6437)
  arc A1631 (79.3496, 41.455) -> (79.2988, 41.455) centre (79.3242, 41.455) ccw
  arc A1632 (78.1812, 40.4589) -> (78.1304, 40.4589) centre (78.1558, 40.4589) ccw
  arc A1633 (81.8642, 38.7237) -> (81.8642, 38.7745) centre (81.8642, 38.7491) ccw
  arc A1634 (80.6835, 38.1222) -> (80.7081, 38.0778) centre (80.6958, 38.1) ccw
  arc A1635 (81.2405, 37.5299) -> (81.1897, 37.5299) centre (81.2151, 37.5299) ccw
  arc A1636 (81.6046, 36.8808) -> (81.8642, 37.1404) centre (81.6046, 37.1404) ccw
  arc A1637 (78.4154, 39.9142) -> (78.4154, 39.965) centre (78.4154, 39.9396) ccw
  arc A1638 (80.6704, 39.6437) -> (80.7212, 39.6437) centre (80.6958, 39.6437) ccw
  line L492 (81.8642, 39.6437) -> (81.8642, 39.3192)
  arc A1639 (81.2151, 37.5553) -> (81.2151, 37.5045) centre (81.2151, 37.5299) ccw
  line L493 (81.8642, 39.3192) -> (80.6958, 39.3192)
  line L494 (81.8642, 38.7491) -> (80.6958, 38.7491)
  arc A1640 (80.9554, 36.8554) -> (80.9554, 36.9062) centre (80.9554, 36.8808) ccw
  line L495 (80.6958, 38.1) -> (81.8642, 38.7491)
  arc A1641 (78.1558, 40.9612) -> (78.1558, 40.9104) centre (78.1558, 40.9358) ccw
  arc A1642 (79.3242, 40.9104) -> (79.3242, 40.9612) centre (79.3242, 40.9358) ccw
  arc A1643 (81.6046, 36.8554) -> (81.6046, 36.9062) centre (81.6046, 36.8808) ccw
  line L496 (81.8642, 38.1) -> (80.6958, 38.1)
  line L497 (78.1558, 40.1992) -> (78.1558, 40.4589)
  arc A1644 (80.7212, 39.6437) -> (80.6704, 39.6437) centre (80.6958, 39.6437) ccw
  arc A1645 (81.0204, 39.9683) -> (80.6958, 39.6437) centre (81.0204, 39.6437) ccw
  arc A1646 (81.8388, 37.1404) -> (81.8896, 37.1404) centre (81.8642, 37.1404) ccw
  line L498 (81.2151, 37.3352) -> (81.2151, 37.5299)
  arc A1647 (81.8388, 39.3192) -> (81.8896, 39.3192) centre (81.8642, 39.3192) ccw
  arc A1648 (79.0646, 39.9142) -> (79.0646, 39.965) centre (79.0646, 39.9396) ccw
  arc A1649 (81.6046, 36.9062) -> (81.6046, 36.8554) centre (81.6046, 36.8808) ccw
  arc A1650 (78.4154, 38.8959) -> (78.4154, 38.8451) centre (78.4154, 38.8705) ccw
  arc A1651 (79.0646, 39.5125) -> (79.0646, 39.4617) centre (79.0646, 39.4871) ccw
  arc A1652 (78.6203, 39.0124) -> (78.6649, 38.9881) centre (78.6426, 39.0003) ccw
  arc A1653 (80.6958, 37.1404) -> (80.9554, 36.8808) centre (80.9554, 37.1404) ccw
  arc A1654 (73.8152, 37.6597) -> (73.7644, 37.6597) centre (73.7898, 37.6597) ccw
  arc A1655 (78.4154, 39.965) -> (78.4154, 39.9142) centre (78.4154, 39.9396) ccw
  line L499 (79.3242, 40.9358) -> (79.3242, 41.455)
  arc A1656 (79.3496, 40.4589) -> (79.2988, 40.4589) centre (79.3242, 40.4589) ccw
  arc A1657 (80.7212, 37.5299) -> (80.6704, 37.5299) centre (80.6958, 37.5299) ccw
  line L500 (73.7898, 36.8808) -> (73.7898, 37.6597)
  arc A1658 (81.8388, 39.6437) -> (81.8896, 39.6437) centre (81.8642, 39.6437) ccw
  arc A1659 (80.6958, 39.3446) -> (80.6958, 39.2938) centre (80.6958, 39.3192) ccw
  line L501 (81.8642, 37.5299) -> (81.8642, 37.1404)
  arc A1660 (81.5396, 39.9429) -> (81.5396, 39.9937) centre (81.5396, 39.9683) ccw
  arc A1661 (4.0462, 47.7012) -> (3.9954, 47.7012) centre (4.0208, 47.7012) ccw
  arc A1662 (5.5307, 46.5074) -> (5.5307, 46.5582) centre (5.5307, 46.5328) ccw
  arc A1663 (80.6958, 38.1254) -> (80.6958, 38.0746) centre (80.6958, 38.1) ccw
  line L502 (80.6958, 37.1404) -> (80.6958, 37.5299)
  line L503 (73.0758, 38.1649) -> (73.0758, 38.814)
  line L504 (73.0758, 39.243) -> (74.2442, 39.6325)
  arc A1664 (73.5697, 38.1649) -> (73.6205, 38.1649) centre (73.5951, 38.1649) ccw
  arc A1665 (74.2188, 38.5544) -> (74.2696, 38.5544) centre (74.2442, 38.5544) ccw
  arc A1666 (2.8448, 47.7266) -> (2.8448, 47.6758) centre (2.8448, 47.7012) ccw
  line L505 (3.1694, 47.0521) -> (2.8448, 47.0521)
  arc A1667 (73.0758, 38.1903) -> (73.0758, 38.1395) centre (73.0758, 38.1649) ccw
  arc A1668 (73.8547, 38.8394) -> (73.8547, 38.7886) centre (73.8547, 38.814) ccw
  arc A1669 (73.9846, 38.7886) -> (73.9846, 38.8394) centre (73.9846, 38.814) ccw
  arc A1670 (3.1694, 47.0521) -> (3.1694, 47.7012) centre (3.1694, 47.3767) ccw
  arc A1671 (3.1694, 47.7266) -> (3.1694, 47.6758) centre (3.1694, 47.7012) ccw
  arc A1672 (2.8448, 47.0775) -> (2.8448, 47.0267) centre (2.8448, 47.0521) ccw
  line L506 (74.2442, 39.6325) -> (73.0758, 40.0219)
  arc A1673 (73.4004, 37.2957) -> (73.4004, 37.2449) centre (73.4004, 37.2703) ccw
  arc A1674 (81.0204, 39.9429) -> (81.0204, 39.9937) centre (81.0204, 39.9683) ccw
  arc A1675 (4.5401, 47.6758) -> (4.5401, 47.7266) centre (4.5401, 47.7012) ccw
  arc A1676 (4.4103, 47.1565) -> (4.4103, 47.2073) centre (4.4103, 47.1819) ccw
  arc A1677 (2.8702, 47.7012) -> (2.8194, 47.7012) centre (2.8448, 47.7012) ccw
  arc A1678 (3.1694, 47.0775) -> (3.1694, 47.0267) centre (3.1694, 47.0521) ccw
  line L507 (5.0114, 46.5328) -> (5.5307, 46.5328)
  arc A1679 (78.1812, 40.1992) -> (78.1304, 40.1992) centre (78.1558, 40.1992) ccw
  arc A1680 (4.0208, 47.7266) -> (4.0208, 47.6758) centre (4.0208, 47.7012) ccw
  line L508 (4.5401, 46.5328) -> (4.0208, 46.5328)
  line L509 (74.1793, 37.2703) -> (73.4004, 37.2703)
  arc A1681 (73.9846, 38.8394) -> (73.9846, 38.7886) centre (73.9846, 38.814) ccw
  arc A1682 (74.2362, 39.6084) -> (74.2522, 39.6566) centre (74.2442, 39.6325) ccw
  arc A1683 (73.8547, 38.7886) -> (73.8547, 38.8394) centre (73.8547, 38.814) ccw
  arc A1684 (80.6704, 39.3192) -> (80.7212, 39.3192) centre (80.6958, 39.3192) ccw
  arc A1685 (81.0204, 39.9937) -> (81.0204, 39.9429) centre (81.0204, 39.9683) ccw
  arc A1686 (73.1012, 38.814) -> (73.0504, 38.814) centre (73.0758, 38.814) ccw
  arc A1687 (3.9954, 46.5328) -> (4.0462, 46.5328) centre (4.0208, 46.5328) ccw
  line L510 (4.0208, 46.5328) -> (4.0208, 47.7012)
  arc A1688 (3.257, 47.0634) -> (3.2115, 47.0407) centre (3.2343, 47.0521) ccw
  arc A1689 (74.2442, 38.5544) -> (73.9846, 38.814) centre (73.9846, 38.5544) ccw
  arc A1690 (3.4712, 46.5214) -> (3.5166, 46.5442) centre (3.4939, 46.5328) ccw
  arc A1691 (73.0838, 40.046) -> (73.0678, 39.9978) centre (73.0758, 40.0219) ccw
  arc A1692 (3.1694, 47.0267) -> (3.1694, 47.0775) centre (3.1694, 47.0521) ccw
  arc A1693 (2.8194, 46.5328) -> (2.8702, 46.5328) centre (2.8448, 46.5328) ccw
  line L511 (74.2442, 38.1649) -> (74.2442, 38.5544)
  line L512 (4.0208, 47.7012) -> (4.5401, 47.7012)
  arc A1694 (74.1793, 37.2449) -> (74.1793, 37.2957) centre (74.1793, 37.2703) ccw
  arc A1695 (74.2188, 38.1649) -> (74.2696, 38.1649) centre (74.2442, 38.1649) ccw
  arc A1696 (73.8547, 38.814) -> (73.5951, 38.5544) centre (73.8547, 38.5544) ccw
  arc A1697 (4.5401, 46.5074) -> (4.5401, 46.5582) centre (4.5401, 46.5328) ccw
  line L513 (81.0204, 39.9683) -> (81.5396, 39.9683)
  line L514 (2.8448, 47.7012) -> (3.1694, 47.7012)
  arc A1698 (80.9554, 36.9062) -> (80.9554, 36.8554) centre (80.9554, 36.8808) ccw
  line L515 (81.2151, 37.5299) -> (81.8642, 37.5299)
  arc A1699 (4.0208, 47.2073) -> (4.0208, 47.1565) centre (4.0208, 47.1819) ccw
  arc A1700 (5.0368, 47.7012) -> (4.986, 47.7012) centre (5.0114, 47.7012) ccw
  arc A1701 (74.2696, 38.5544) -> (74.2188, 38.5544) centre (74.2442, 38.5544) ccw
  arc A1702 (73.5697, 38.5544) -> (73.6205, 38.5544) centre (73.5951, 38.5544) ccw
  arc A1703 (73.6205, 38.5544) -> (73.5697, 38.5544) centre (73.5951, 38.5544) ccw
  arc A1704 (74.2522, 39.6084) -> (74.2362, 39.6566) centre (74.2442, 39.6325) ccw
  arc A1705 (5.0114, 46.5582) -> (5.0114, 46.5074) centre (5.0114, 46.5328) ccw
  line L516 (4.0208, 47.1819) -> (4.4103, 47.1819)
  arc A1706 (73.5951, 38.1395) -> (73.5951, 38.1903) centre (73.5951, 38.1649) ccw
  arc A1707 (73.0504, 38.1649) -> (73.1012, 38.1649) centre (73.0758, 38.1649) ccw
  line L517 (3.4939, 46.5328) -> (3.2343, 47.0521)
  arc A1708 (4.0208, 46.5582) -> (4.0208, 46.5074) centre (4.0208, 46.5328) ccw
  arc A1709 (21.0058, 53.8311) -> (21.0058, 53.7803) centre (21.0058, 53.8057) ccw
  arc A1710 (22.1865, 55.0605) -> (22.1619, 55.1049) centre (22.1742, 55.0827) ccw
  arc A1711 (18.8327, 52.4482) -> (18.8835, 52.4482) centre (18.8581, 52.4482) ccw
  arc A1712 (18.8835, 52.6429) -> (18.8327, 52.6429) centre (18.8581, 52.6429) ccw
  arc A1713 (5.9941, 46.8503) -> (5.9941, 46.7995) centre (5.9941, 46.8249) ccw
  arc A1714 (7.4084, 47.1641) -> (7.4499, 47.1348) centre (7.4292, 47.1495) ccw
  line L518 (5.0114, 47.7012) -> (5.0114, 46.5328)
  line L519 (73.9846, 38.814) -> (73.8547, 38.814)
  line L520 (22.1742, 52.8913) -> (21.0058, 53.2807)
  arc A1715 (20.9804, 53.6758) -> (21.0312, 53.6758) centre (21.0058, 53.6758) ccw
  arc A1716 (21.0058, 55.1081) -> (21.0058, 55.0573) centre (21.0058, 55.0827) ccw
  arc A1717 (5.8726, 46.5408) -> (5.9208, 46.5248) centre (5.8967, 46.5328) ccw
  line L521 (18.8581, 52.4482) -> (18.8581, 52.6429)
  arc A1718 (22.1742, 54.4082) -> (22.1742, 54.459) centre (22.1742, 54.4336) ccw
  line L522 (19.2476, 51.9938) -> (18.5984, 51.9938)
  arc A1719 (7.4084, 47.1348) -> (7.4499, 47.1641) centre (7.4291, 47.1494) ccw
  line L523 (21.0058, 52.5018) -> (22.1742, 52.8913)
  arc A1720 (7.8394, 47.6866) -> (7.7979, 47.7158) centre (7.8187, 47.7012) ccw
  line L524 (7.4292, 46.5328) -> (7.4292, 47.1495)
  arc A1721 (7.4546, 47.1495) -> (7.4038, 47.1495) centre (7.4292, 47.1495) ccw
  arc A1722 (22.1742, 55.0573) -> (22.1742, 55.1081) centre (22.1742, 55.0827) ccw
  arc A1723 (18.3642, 52.2534) -> (18.3134, 52.2534) centre (18.3388, 52.2534) ccw
  arc A1724 (19.4818, 52.2534) -> (19.5326, 52.2534) centre (19.5072, 52.2534) ccw
  arc A1725 (19.5326, 52.2534) -> (19.4818, 52.2534) centre (19.5072, 52.2534) ccw
  arc A1726 (18.3642, 52.6429) -> (18.3134, 52.6429) centre (18.3388, 52.6429) ccw
  arc A1727 (22.1996, 53.9355) -> (22.1488, 53.9355) centre (22.1742, 53.9355) ccw
  line L525 (7.4292, 47.1495) -> (7.8187, 47.7012)
  arc A1728 (4.986, 46.5328) -> (5.0368, 46.5328) centre (5.0114, 46.5328) ccw
  arc A1729 (20.9935, 54.4558) -> (21.0181, 54.4114) centre (21.0058, 54.4336) ccw
  arc A1730 (21.0138, 53.3048) -> (20.9978, 53.2566) centre (21.0058, 53.2807) ccw
  arc A1731 (19.2476, 51.9684) -> (19.2476, 52.0192) centre (19.2476, 51.9938) ccw
  arc A1732 (6.3103, 47.7092) -> (6.2621, 47.6932) centre (6.2862, 47.7012) ccw
  arc A1733 (19.2476, 51.9938) -> (19.5072, 52.2534) centre (19.2476, 52.2534) ccw
  line L526 (73.5951, 38.5544) -> (73.5951, 38.1649)
  line L527 (73.5951, 38.1649) -> (73.0758, 38.1649)
  arc A1734 (18.3134, 52.2534) -> (18.3642, 52.2534) centre (18.3388, 52.2534) ccw
  line L528 (6.5783, 46.8249) -> (5.9941, 46.8249)
  line L529 (7.0397, 47.7012) -> (7.4292, 47.1495)
  line L530 (18.3388, 52.2534) -> (18.3388, 52.6429)
  arc A1735 (21.0312, 53.9355) -> (20.9804, 53.9355) centre (21.0058, 53.9355) ccw
  arc A1736 (18.8581, 52.6683) -> (18.8581, 52.6175) centre (18.8581, 52.6429) ccw
  line L531 (18.8581, 52.6429) -> (19.5072, 52.6429)
  arc A1737 (22.1488, 53.6758) -> (22.1996, 53.6758) centre (22.1742, 53.6758) ccw
  line L532 (22.1742, 55.0827) -> (21.0058, 55.0827)
  line L533 (21.0058, 53.8057) -> (22.1742, 53.8057)
  line L534 (5.8967, 46.5328) -> (6.2862, 47.7012)
  line L535 (21.0058, 53.6758) -> (21.0058, 53.9355)
  arc A1738 (3.1694, 47.6758) -> (3.1694, 47.7266) centre (3.1694, 47.7012) ccw
  line L536 (19.5072, 52.6429) -> (19.5072, 52.2534)
  arc A1739 (20.9978, 52.5259) -> (21.0138, 52.4777) centre (21.0058, 52.5018) ccw
  arc A1740 (73.7644, 36.8808) -> (73.8152, 36.8808) centre (73.7898, 36.8808) ccw
  arc A1741 (19.2476, 52.0192) -> (19.2476, 51.9684) centre (19.2476, 51.9938) ccw
  arc A1742 (6.5783, 46.7995) -> (6.5783, 46.8503) centre (6.5783, 46.8249) ccw
  line L537 (2.8448, 46.5328) -> (2.8448, 47.7012)
  arc A1743 (18.5984, 52.0192) -> (18.5984, 51.9684) centre (18.5984, 51.9938) ccw
  line L538 (6.2862, 47.7012) -> (6.6757, 46.5328)
  arc A1744 (21.0058, 54.459) -> (21.0058, 54.4082) centre (21.0058, 54.4336) ccw
  arc A1745 (19.5326, 52.6429) -> (19.4818, 52.6429) centre (19.5072, 52.6429) ccw
  line L539 (22.1742, 54.4336) -> (21.0058, 54.4336)
  arc A1746 (18.5984, 51.9684) -> (18.5984, 52.0192) centre (18.5984, 51.9938) ccw
  arc A1747 (73.0678, 39.2671) -> (73.0838, 39.2189) centre (73.0758, 39.243) ccw
  arc A1748 (19.5072, 52.6175) -> (19.5072, 52.6683) centre (19.5072, 52.6429) ccw